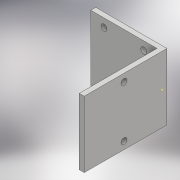
# Autodesk Inventor part: 连接架
Saved by Autodesk Inventor 2017 (Build 210142000, 142)
## iProperties
Part Number: 连接架
Material: 常规
Document SubType Name: 钣金
Designer: PANDA
Density: 1 g/cm^3
Sheet Metal Rule: 默认_mm
Appearance: 默认
Author: PANDA
Autodesk Inventor part; units mm, degrees
ref_plane "YZ Plane" through (0, 0, 0) normal (1, 0, 0) x (0, 1, 0)
ref_plane "XZ Plane" through (0, 0, 0) normal (0, 1, 0) x (-1, 0, 0)
ref_plane "XY Plane" through (0, 0, 0) normal (0, 0, 1) x (1, 0, 0)
sketch "草图1" plane through (0, 0, 0) normal (0, 1, 0) x (-1, 0, 0)
  line L0 (20, 20) -> (-20, 20)
  line L1 (-20, 20) -> (-20, -20)
  line L2 (-20, -20) -> (20, -20)
  line L3 (20, -20) -> (20, 20)
  point P0 (0, 0)
  dimension "d0" = 40
  dimension "d1" = 40
  constraints: 8 end point, 2 parallel, 1 horizontal, 1 perpendicular
  measures "d0" distance of L2.end L1.end
  measures "d1" distance of L1.end L0.end
extrude "拉伸1" add sketch "草图1" along normal blind 3
sketch "草图6" plane through (20, 0, 20) normal (1, 0, 0) x (0, 0, -1)
  point P0 (20, 0)
sketch "草图7" plane through (20, 0, 20) normal (1, 0, 0) x (0, 0, -1)
  line L0 (40, 3) -> (0, 3) projected
  line L1 (0, 0) -> (40, 0)
  line L2 (40, 0) -> (40, 3)
  line L3 (40, 3) -> (0, 3)
  line L4 (0, 3) -> (0, 0)
  point P0 (20, 0)
  constraints: 8 end point, 2 parallel, 1 horizontal, 1 perpendicular
extrude "拉伸6" add sketch "草图7" along normal blind 3
sketch "草图8" plane through (0, 0, 0) normal (0, -1, 0) x (1, 0, 0)
  line L0 (23, -20) -> (23, 20) projected
  line L1 (20, 20) -> (23, 20)
  line L2 (23, 20) -> (23, -20)
  line L3 (23, -20) -> (20, -20)
  line L4 (20, -20) -> (20, 20)
  point P0 (0, 0)
  constraints: 8 end point, 2 parallel, 1 horizontal, 1 perpendicular
extrude "拉伸7" add sketch "草图8" along normal blind 47
sketch "草图9" plane through (23, 0, 20) normal (1, 0, 0) x (0, 0, -1)
  point P0 (20, 0)
sketch "草图10" plane through (23, 0, 20) normal (1, 0, 0) x (0, 0, -1)
  circle A0 centre (35.5, -23) radius 1.8
  point P0 (20, 0)
  dimension "d20" = 3.6
  constraints: 1 centre point
  measures "d20" diameter of A0
extrude "拉伸8" cut sketch "草图10" against normal through all
sketch "草图11" plane through (23, 0, 20) normal (1, 0, 0) x (0, 0, -1)
  circle A0 centre (4.5, -23) radius 1.8
  point P0 (20, 0)
  dimension "d23" = 3.6
  constraints: 1 centre point
  measures "d23" diameter of A0
extrude "拉伸9" cut sketch "草图11" against normal through all
sketch "草图12" plane through (0, 3, 0) normal (0, 1, 0) x (1, 0, 0)
  circle A0 centre (12, 15) radius 1.8
  point P0 (0, 0)
  dimension "d26" = 3.6
  constraints: 1 centre point
  measures "d26" diameter of A0
extrude "拉伸10" cut sketch "草图12" against normal through all
sketch "草图13" plane through (0, 3, 0) normal (0, 1, 0) x (1, 0, 0)
  circle A0 centre (-12, 15) radius 1.8
  point P0 (0, 0)
  dimension "d29" = 3.6
  constraints: 1 centre point
  measures "d29" diameter of A0
extrude "拉伸11" cut sketch "草图13" against normal through all
sketch "草图14" plane through (0, 3, 0) normal (0, 1, 0) x (1, 0, 0)
  circle A0 centre (-12, -15) radius 1.8
  point P0 (0, 0)
  dimension "d32" = 3.6
  constraints: 1 centre point
  measures "d32" diameter of A0
extrude "拉伸12" cut sketch "草图14" against normal through all
sketch "草图15" plane through (0, 3, 0) normal (0, 1, 0) x (1, 0, 0)
  circle A0 centre (12, -15) radius 1.8
  point P0 (0, 0)
  dimension "d35" = 3.6
  constraints: 1 centre point
  measures "d35" diameter of A0
extrude "拉伸13" cut sketch "草图15" against normal through all
equation "\"折弯半径\" = 厚度"
equation "\"折弯释压宽度\" = 厚度"
equation "\"折弯释压深度\" = 0.5 * 厚度"
equation "\"拐角释压尺寸\" = 4 * 厚度"
equation "\"最小余量\" = 2 * 厚度"
equation "\"过渡半径\" = 折弯半径"
equation "\"Jacobi半径尺寸\" = 折弯半径"
equation "\"间隙大小\" = 厚度"
equation "\"厚度\" = 0.5"
